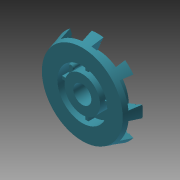
# Autodesk Inventor part: Kornylak- Half Wheel
Saved by Autodesk Inventor 2014 (Build 180170000, 170)
## iProperties
Created: 2014-02-03
Part Number: Kornylak- Half Wheel
Material: Generic
Document SubType Name: Modeling
Designer: Spooner
Density: 1 g/cm^3
Appearance: Cadet Blue
Mass: 7.88239 g
Surface Area: 62.3594 cm^2
Volume: 7.88239 cm^3
Author: Spooner
Autodesk Inventor part; units mm, degrees
ref_plane "YZ Plane" through (0, 0, 0) normal (1, 0, 0) x (0, 1, 0)
ref_plane "XZ Plane" through (0, 0, 0) normal (0, 1, 0) x (-1, 0, 0)
sketch "Sketch14" plane through (0, 0, 0) normal (0, 0, 1) x (1, 0, 0)
  circle A0 centre (0, 0) radius 21.971
  dimension "d60" = 43.942
  constraints: 1 centre point, 1 coincident
  measures "d60" diameter of A0
ref_plane "Work Plane4" through (0, 0, -8.3185) normal (0, 0, 1) x (1, 0, 0)
sketch "Sketch15" plane through (0, 0, -8.3185) normal (0, 0, 1) x (1, 0, 0)
  circle A0 centre (0, 0) radius 24.511
  dimension "d62" = 49.022
  constraints: 1 centre point, 1 coincident
  measures "d62" diameter of A0
loft "Loft3" add profiles "Sketch14", "Sketch15"
sketch "Sketch16" plane through (0, 0, 0) normal (0, 0, 1) x (1, 0, 0)
  circle A0 centre (0, 0) radius 21.971 projected
  circle A1 centre (0, 0) radius 4.8895
  dimension "d67" = 9.779
  constraints: 1 centre point, 1 coincident
  measures "d67" diameter of A1
extrude "Extrusion9" cut sketch "Sketch16" against normal through all contours A1
sketch "Sketch17" plane through (0, 0, 0) normal (0, 0, 1) x (1, 0, 0)
  circle A0 centre (0, 0) radius 21.971 projected
  circle A1 centre (0, 0) radius 9.652
  circle A2 centre (0, 0) radius 13.5255
  dimension "d70" = 27.051
  dimension "d71" = 19.304
  constraints: 2 centre point, 2 coincident
  measures "d70" diameter of A2
  measures "d71" diameter of A1
extrude "Extrusion10" cut sketch "Sketch17" against normal blind 5.969 contours A2
sketch "Sketch18" plane through (0, 0, -5.969) normal (0, 0, 1) x (1, 0, 0)
  circle A0 centre (0, 0) radius 9.652 projected
  circle A1 centre (0, 0) radius 13.5255 projected
  line L0 (-0.7937, 13.5022) -> (-0.7937, 9.6193)
  line L1 (0.7938, 13.5022) -> (0.7938, 9.6193)
  arc A2 (0.7938, 13.5022) -> (-0.7937, 13.5022) centre (0, 0) ccw
  arc A3 (0.7938, 9.6193) -> (-0.7937, 9.6193) centre (0, 0) ccw
  dimension "d74" = 1.5875
  constraints: 8 point on circle, 4 end point, 2 centre point, 2 concentric, 2 parallel, 1 vertical
  measures "d74" distance between parallel lines of L1 L0
extrude "Extrusion11" add sketch "Sketch18" along normal blind 3.4925 contours A0 L0 A1 L1 picked at (0.6175, 10.9233)
pattern_circular "Circular Pattern3" count 4 over 360 about axis through (0, 0, 0) along (0, 0, -1) of "Extrusion11"
sketch "Sketch19" plane through (0, 0, -5.969) normal (0, 0, 1) x (1, 0, 0)
  arc A0 (-0.7937, 9.6193) -> (-9.6193, 0.7938) centre (0, 0) ccw projected
  line L0 (-0.7937, 9.6193) -> (-0.7937, 13.5022) projected
  arc A1 (-0.7937, 13.5022) -> (-13.5022, 0.7938) centre (0, 0) ccw projected
  circle A2 centre (-6.1658, 9.8123) radius 1.5748
  dimension "d80" = 3.1496
  dimension "d85" = 3.7973
  dimension "d86" = 0.3619
  dimension "d87" = 0.3619
  constraints: 1 centre point
  measures "d80" diameter of A2
  measures "d85" distance edge to line of A2 L0
extrude "Extrusion12" add sketch "Sketch19" along normal up to surface (5.969 mm away)
chamfer "Chamfer1" distance 0.508 angle 45 1 edges at (-7.7406, 9.8123, 0)
sketch "Sketch20" plane through (0, 0, -8.3185) normal (0, 0, -1) x (-1, 0, 0)
  circle A0 centre (0, 0) radius 4.8895 projected
  circle A1 centre (0, 0) radius 24.511 projected
  line L0 (-0.7938, 13.5022) -> (-0.7938, 9.6193) projected
  line L1 (0.7937, 9.6193) -> (0.7937, 13.5022) projected
  line L2 (0.1231, 16.8906) -> (3.1931, 24.3021)
  line L3 (11.8564, 12.0305) -> (14.9264, 19.442)
  arc A2 (11.8564, 12.0305) -> (0.1231, 16.8906) centre (0, 0) ccw
  line L4 (0, 0) -> (12.7281, 30.7284) construction
  line L5 (0, 0) -> (0, 30.7704) construction
  dimension "d93" = 22.5
  dimension "d94" = 6.35
  dimension "d95" = 6.35
  dimension "d96" = 6.35
  dimension "d97" = 6.35
  dimension "d98" = 7.62
  constraints: 8 end point, 4 point on circle, 1 centre point, 1 coincident, 1 concentric, 1 parallel
  measures "d93" angle of L4 L5
  measures "d94" distance from line of L4 L2.end
  measures "d95" distance from line of L4 L3.end
  measures "d96" distance from line of L4 L2.start
  measures "d97" distance from line of L4 L3.start
  measures "d98" radial gap between concentric circles of A2 A1
extrude "Extrusion13" cut sketch "Sketch20" against normal blind 5.842 contours L3 A2 L2 A1 picked at (11.8597, 18.4203)
sketch "Sketch21" plane through (0, 0, -8.3185) normal (0, 0, -1) x (-0.9238795, -0.3826834, 0)
  line L0 (-6.35, 15.6519) -> (-6.35, 23.6742) projected
  line L1 (6.35, 23.6742) -> (6.35, 15.6519) projected
  line L2 (-6.35, 21.1342) -> (-6.985, 21.1342)
  line L3 (-6.985, 21.1342) -> (-6.985, 20.4992)
  line L4 (-6.985, 20.4992) -> (-6.35, 20.4992)
  line L5 (-6.35, 20.4992) -> (-6.35, 21.1342)
  line L6 (6.35, 21.1342) -> (6.985, 21.1342)
  line L7 (6.985, 21.1342) -> (6.985, 20.4992)
  line L8 (6.985, 20.4992) -> (6.35, 20.4992)
  line L9 (6.35, 20.4992) -> (6.35, 21.1342)
  point P0 (-6.6675, 21.1342)
  point P1 (6.6675, 21.1342)
  point P2 (-6.6675, 20.4992)
  point P3 (6.6675, 20.4992)
  dimension "d101" = 0.635
  dimension "d102" = 0.635
  dimension "d103" = 0.635
  dimension "d104" = 2.54
  constraints: 16 end point, 4 midpoint, 4 parallel, 2 horizontal, 2 horizontal alignment, 2 perpendicular, 2 point on line
  measures "d101" distance between parallel lines of L4 L2
  measures "d102" distance between parallel lines of L5 L3
  measures "d103" distance between parallel lines of L1 L7
  measures "d104" distance of L2.start L0.end
revolve "Revolution2" cut sketch "Sketch21" angle 360 about axis through (-1.3914, 21.6118, -8.3185) along (-0.9238795, -0.3826834, 0)
pattern_circular "Circular Pattern4" count 8 over 360 about axis through (0, 0, -8.3185) along (0, 0, 1) of "Extrusion13", "Revolution2"
equation "\"d86\" = d87"
equation "\"d94\" = d95"
equation "\"d96\" = d95"
equation "\"d97\" = d96"
equation "\"d103\" = d102"
body "Solid2"
